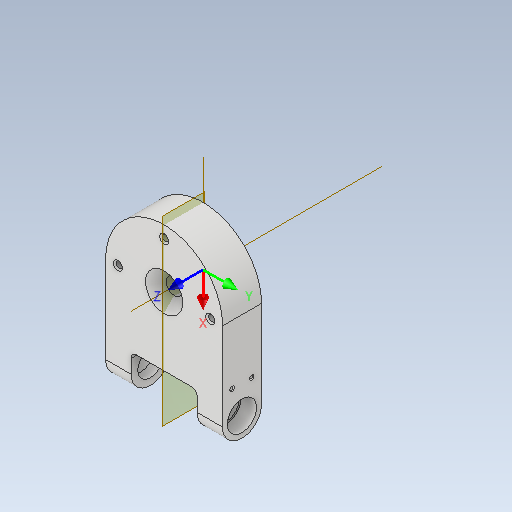
# Autodesk Inventor part: Shoulder_Joint_v2
Saved by Autodesk Inventor 2021.4 (Build 254397000, 397)
## iProperties
Created: 2020-05-04
Part Number: Shoulder_Joint_v2
Material: PVC-Piping
Document SubType Name: Modeling
Designer: Alex
Density: 1.4 g/cm^3
Appearance: Smooth - White
Mass: 89.3584 g
Surface Area: 161.384 cm^2
Volume: 63.8274 cm^3
SJ_D_out: 60,000 mm
Author: Alex
Autodesk Inventor part; units mm, degrees
ref_plane "YZ Plane" through (0, 0, 0) normal (1, 0, 0) x (0, 1, 0)
sketch "Skizze1" plane through (0, 0, 0) normal (0, 0, 1) x (1, 0, 0)
  arc A0 (30, 0) -> (-30, 0) centre (0, 0) ccw
  line L0 (-17, -35) -> (-17, -55)
  line L1 (-17, -55) -> (-30, -55)
  line L2 (-30, -55) -> (-30, 0)
  line L3 (0, 0) -> (0, 30) construction
  line L4 (17, -35) -> (17, -55)
  line L5 (17, -55) -> (30, -55)
  line L6 (30, -55) -> (30, 0)
  line L7 (-17, -35) -> (17, -35)
  dimension "SJ_D_out" = 60
  dimension "d1" = 55
  dimension "d2" = 17
  dimension "d3" = 35
  dimension "d34" = 13
  constraints: 16 end point, 4 symmetric about line, 3 point on circle, 2 horizontal, 2 vertical, 1 centre point, 1 coincident, 1 parallel, 1 tangent
  measures "SJ_D_out" diameter of A0
  measures "d1" distance from line of L1 point (0, 0)
  measures "d2" distance from line of L0 point (0, 0)
  measures "d3" distance from line of L7 point (0, 0)
  measures "d34" distance of L0.end L1.end
extrude "Grundform" add sketch "Skizze1" along normal blind 20
fillet "Konturverrundungen" radius 10 4 edges at (-23.5, -55, 20) (23.5, -55, 20) (-23.5, -55, 0) (23.5, -55, 0)
fillet "Konturverrundungen" radius 3 2 edges at (-17, -35, 10) (17, -35, 10)
ref_plane "Konstruktionshilfsebene" through (0, 0, 0) normal (0, -1, 0) x (1, 0, 0)
ref_plane "Arbeitsebene1" through (0, 30, 0) normal (0, -1, 0) x (1, 0, 0)
sketch "Skizze2" plane through (0, 0, 0) normal (0, -1, 0) x (1, 0, 0)
  line L0 (-30, 0) -> (-17, 0) construction
  line L1 (-18, 0) -> (-18, 10)
  line L2 (-17, 20) -> (-17, 0) construction
  line L3 (-18, 10) -> (0, 10)
  line L4 (0, 10) -> (0, 0)
  line L5 (-17, 0) -> (-14, 0) construction
  line L6 (-18, 0) -> (0, 0)
  dimension "d11" = 36
  dimension "d12" = 10
  constraints: 8 end point, 1 horizontal, 1 perpendicular, 1 point on line, 1 vertical
  measures "d11" diameter of L1 L4
  measures "d12" distance between parallel lines of L0 L3
revolve "Wellenaufnahme" cut sketch "Skizze2" angle 360 about axis through (0, 0, 10) along (0, 0, -1)
sketch "Skizze3" plane through (0, 0, 20) normal (0, 0, 1) x (1, 0, 0)
  point P0 (0, 0)
  point P1 (0, 0)
  constraints: 1 coincident
hole "Senkung für M8 Innensechskantschraube" at (0, 0, 20) direction (0, 0, -1) diameter 8.4 end through all countersink diameter 19 countersink angle 90 clearance for "Innensechskant-Senkkopfschraube DIN EN ISO 10642" size "M8" standard "DIN"
ref_plane "Konstruktionshilfsebene:2" through (0, 0, 10) normal (0, 0, -1) x (-1, 0, 0)
sketch "Skizze4" plane through (0, 0, 10) normal (0, 0, -1) x (-1, 0, 0)
  line L0 (-30, -45) -> (-30, 0) construction
  line L1 (-17, -38.5) -> (-17, -45)
  line L2 (-30, -45) -> (-17, -45) projected
  line L3 (-17, -45) -> (-30, -45)
  line L4 (-30, -45) -> (-30, -37.5)
  line L5 (0, 0) -> (0, -35) construction
  line L6 (14, -35) -> (-14, -35) construction
  line L7 (-17, -38) -> (-17, -45) construction
  line L8 (42, -45) -> (-42, -45) construction
  line L9 (-30, -37.5) -> (-22, -37.5)
  line L10 (-22, -37.5) -> (-22, -38.5)
  line L11 (-22, -38.5) -> (-17, -38.5)
  line L12 (17, -38.5) -> (17, -45)
  line L13 (30, -45) -> (17, -45)
  line L14 (17, -45) -> (30, -45)
  line L15 (30, -45) -> (30, -37.5)
  line L16 (30, -37.5) -> (22, -37.5)
  line L17 (22, -37.5) -> (22, -38.5)
  line L18 (22, -38.5) -> (17, -38.5)
  dimension "d35" = 13
  dimension "d39" = 15
  dimension "d40" = 8
  constraints: 28 end point, 7 symmetric about line, 4 perpendicular, 2 collinear, 2 point on line, 1 midpoint
  measures "d35" diameter of L11 L8
  measures "d39" diameter of L9 L2
  measures "d40" distance between parallel lines of L10 L0
revolve "Axial-Radial Nadellager Innenprofil" cut sketch "Skizze4" angle 360 about axis through (8.5, -45, 10) along (1, 0, 0)
sketch "Skizze5" plane through (30, 0, 20) normal (1, 0, 0) x (0, 0, -1)
  circle A0 centre (5, -30.5) radius 1.2 construction
  circle A1 centre (15, -30.5) radius 1.2 construction
  point P0 (20, 0)
  constraints: 2 coincident
hole "Gewinde_Keine_ISO Metrisches Profil_2_Winkel(2)" at (30, -30.5, 15) at (30, -30.5, 5) direction (-1, 0, 0) diameter 1.567 depth 10 tip angle 118 thread size "M2x0.4" class "6H" standard "ISO Metric profile"
ref_plane "Spiegelebene" through (0, 0, 20) normal (1, 0, 0) x (0, 0, -1)
mirror "Gewindebohrung gespiegelt" about plane through (0, 0, 20) normal (1, 0, 0) of "Gewinde_Keine_ISO Metrisches Profil_2_Winkel(2)"
chamfer "Ansenkung Gewindebohrung M2x0,4mm" distance 0.4 angle 45 4 edges at (30, -30.5, 15.7835) (30, -30.5, 5.7835) (-30, -30.5, 15.7835) (-30, -30.5, 5.7835)
sketch "Sketch6" plane through (0, 0, 20) normal (0, 0, 1) x (1, 0, 0)
  circle A0 centre (0, 0) radius 4.2 construction
  circle A1 centre (0, 0) radius 23.75 construction
  circle A2 centre (0, 0) radius 9.5 construction
  line L0 (0, 0) -> (0, 23.75) construction
  line L1 (23.75, 0) -> (-23.75, 0) construction
  line L2 (0, 0) -> (23.75, 0) construction
  dimension "FixHole_Rad" = 23.75
  dimension "FixHole_Side_Angle" = 90
  constraints: 6 end point, 3 point on circle, 2 coincident, 1 centre point, 1 horizontal, 1 vertical
  measures "FixHole_Rad" radius of A1
  measures "FixHole_Side_Angle" angle of L0 L2
hole "Hole3" at (0, 23.75, 20) at (-23.75, 0, 20) at (23.75, 0, 20) direction (0, 0, -1) diameter 3.242 depth 12 tip angle 118 thread size "M4x0.7" class "6H" standard "ISO Metric profile"
chamfer "Chamfer2" distance 0.7 angle 45 3 edges at (-23.75, 1.621, 20) (23.75, 1.621, 20) (0, 25.371, 20)
ref_plane "Arbeitsebene5" through (0, 0, 20) normal (1, 0, 0) x (0, 0, -1)
equation "\"d6\" = 0.5 * d4"
equation "\"d4\" = 20"
